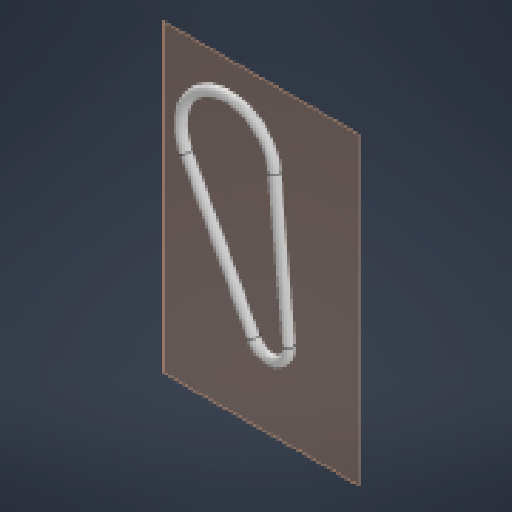
# Autodesk Inventor part: Belt
Saved by Autodesk Inventor 2024.2 (Build 282272000, 272)
## iProperties
Created: 2024-01-10
Part Number: Belt
Material: 一般
Document SubType Name: Modeling
Designer: Hanaoka
Density: 1 g/cm^3
Appearance: 既定
Author: Hanaoka
Autodesk Inventor part; units mm, degrees
ref_plane "YZ Plane" through (0, 0, 0) normal (1, 0, 0) x (0, 1, 0)
ref_plane "XZ Plane" through (0, 0, 0) normal (0, 1, 0) x (-1, 0, 0)
ref_plane "XY Plane" through (0, 0, 0) normal (0, 0, 1) x (1, 0, 0)
ref_plane "作業平面1" through (0, 0, 0) normal (0, 0, 1) x (1, 0, 0)
sketch "スケッチ1" plane through (0, 0, 0) normal (0, 0, 1) x (1, 0, 0)
  circle A0 centre (1.4986, -6.7164) radius 2.5 projected
  circle A1 centre (-2.9986, 8.2164) radius 5.5 projected
  line L0 (2.4745, 8.7597) -> (3.9863, -6.4695)
  line L1 (-7.8615, 5.647) -> (-0.7119, -7.8843)
  arc A2 (1.4794, 8.6609) -> (-6.9773, 6.1141) centre (-2.9986, 8.2164) ccw
  line L2 (1.4794, 8.6609) -> (2.9912, -6.5682)
  arc A3 (0.1723, -7.4172) -> (2.9912, -6.5682) centre (1.4986, -6.7164) ccw
  line L3 (-6.9773, 6.1141) -> (0.1723, -7.4172)
  point P0 (0, 0)
  dimension "d0" = 1
  dimension "d1" = 1
  constraints: 8 end point, 8 point on circle, 8 tangent, 2 centre point, 2 coincident
  measures "d0" radial gap between concentric circles of A2 A1
  measures "d1" radial gap between concentric circles of A0 A3
extrude "押し出し1" add sketch "スケッチ1" along normal blind 1 contours A0 L3 A3 L2 | A0 L2 A1 L0 | L1 A1 L3 A0 | A1 L2 A2 L3 picked at (3.0117, -5.3596) picked at (-6.3062, 4.4531)
fillet "フィレット1" radius 0.5 16 edges at (-4.5846, 13.4828, 1) (-4.2867, -1.1187, 1) (2.2195, -9.1102, 1) (3.2304, 1.1451, 1) (-4.5846, 13.4828, 0) (-4.2867, -1.1187, 0) (2.2195, -9.1102, 0) (3.2304, 1.1451, 0) (1.9311, -8.1527, 1) (-3.4025, -0.6515, 1) (-4.2962, 12.5253, 1) (2.2353, 1.0464, 1) (1.9311, -8.1527, 0) (-3.4025, -0.6515, 0) (-4.2962, 12.5253, 0) (2.2353, 1.0464, 0)
